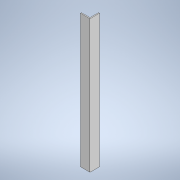
# Autodesk Inventor part: Ugol800
Saved by Autodesk Inventor 2022 (Build 260153000, 153)
## iProperties
Created: 2023-08-15
Part Number: Ugol800
Material: Generic
Document SubType Name: Modeling
Designer: Kippi
Density: 1 g/cm^3
Appearance: Default
Mass: 617.5 g
Surface Area: 2609.5 cm^2
Volume: 617.5 cm^3
Author: Kippi
Autodesk Inventor part; units mm, degrees
ref_plane "YZ Plane" through (0, 0, 0) normal (1, 0, 0) x (0, 1, 0)
ref_plane "XZ Plane" through (0, 0, 0) normal (0, 1, 0) x (-1, 0, 0)
ref_plane "XY Plane" through (0, 0, 0) normal (0, 0, 1) x (1, 0, 0)
sketch "Sketch1" plane through (0, 0, 0) normal (0, 1, 0) x (-1, 0, 0)
  line L0 (38.8889, 27.7778) -> (-11.1111, 27.7778)
  line L1 (-11.1111, 27.7778) -> (-11.1111, -22.2222)
  line L2 (38.8889, 27.7778) -> (38.8889, 22.7778)
  line L3 (38.8889, 22.7778) -> (-6.1111, 22.7778)
  line L4 (-6.1111, 22.7778) -> (-6.1111, -22.2222)
  line L5 (-6.1111, -22.2222) -> (-11.1111, -22.2222)
  point P0 (0, 0)
  dimension "d0" = 50
  dimension "d1" = 50
  dimension "d2" = 5
  dimension "d3" = 5
  constraints: 12 end point, 4 perpendicular, 1 horizontal, 1 vertical
  measures "d0" distance of L0.end L1.end
  measures "d1" distance of L0.start L0.end
  measures "d2" distance of L4.end L1.end
  measures "d3" distance of L0.start L2.end
extrude "Extrusion1" add sketch "Sketch1" along normal blind 700
body "Solid1"
